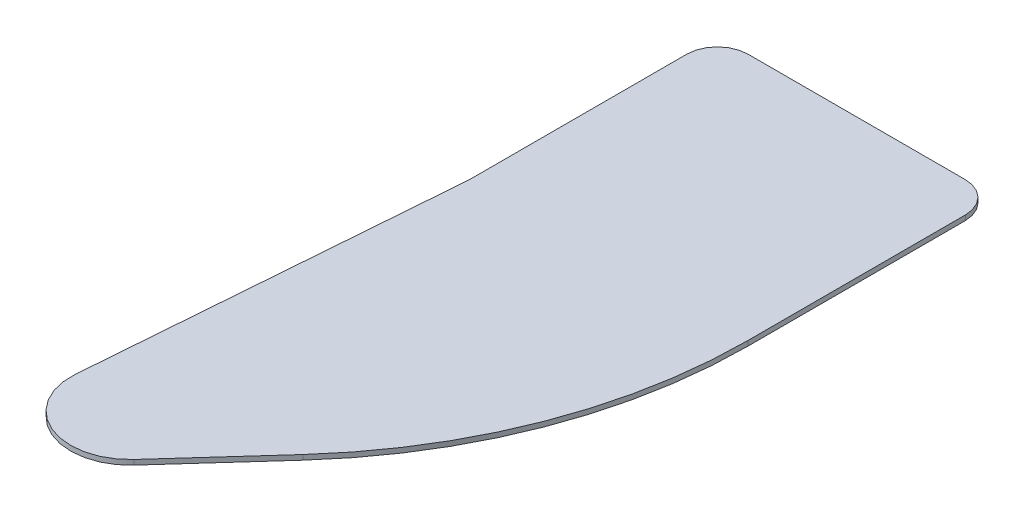
# Autodesk Inventor part: m2stack_bottom_1
Saved by Autodesk Inventor 2026 (Build 300175000, 175)
## iProperties
Created: 2025-05-07
Part Number: m2stack_bottom_1
Material: Generic
Document SubType Name: Modeling
Designer: Paul Juschitz
Density: 1 g/cm^3
Appearance: Default
Author: Paul Juschitz
Autodesk Inventor part; units mm, degrees
ref_plane "YZ Plane" through (0, 0, 0) normal (1, 0, 0) x (0, 1, 0)
ref_plane "XZ Plane" through (0, 0, 0) normal (0, 1, 0) x (-1, 0, 0)
ref_plane "XY Plane" through (0, 0, 0) normal (0, 0, 1) x (1, 0, 0)
sketch "Sketch1" plane through (0, 0, 0) normal (0, 1, 0) x (-1, 0, 0)
  line L0 (50, 0) -> (-50, 0)
  line L1 (0, 50) -> (0, -50)
  line L2 (-25.0156, 15.5413) -> (-25.0156, -28.4587)
  arc A0 (-25.0156, -28.4587) -> (-18.8156, -34.6587) centre (-18.8156, -28.4587) ccw
  line L3 (-18.8156, -34.6587) -> (25.1844, -34.6587)
  arc A1 (25.1844, -34.6587) -> (31.3844, -28.4587) centre (25.1844, -28.4587) ccw
  line L4 (31.3844, -28.4587) -> (31.3844, 15.5413)
  line L5 (31.3844, 15.5413) -> (37.1483, 89.6103)
  arc A2 (37.1483, 89.6103) -> (16.2805, 98.5862) centre (25.1844, 90.5413) ccw
  line L6 (16.2805, 98.5862) -> (0.0171, 80.5862)
  arc A3 (0.0171, 80.5862) -> (-25.0156, 15.5413) centre (72.0072, 15.5413) ccw
  line L7 (31.3844, 15.5413) -> (-25.0156, 15.5413) construction
  point P0 (0, 0)
  point P1 (31.3844, 15.5413)
  dimension "d0" = 100
  dimension "d1" = 100
  dimension "d3" = 56.4
  dimension "d4" = 6.2
  dimension "case_foot_outer_radius" = 12
  dimension "case_foot_width" = 75
  dimension "d7" = 18
  constraints: 16 end point, 8 point on circle, 8 tangent, 4 centre point, 3 perpendicular, 3 vertical, 2 equal length, 2 midpoint, 1 coincident, 1 equal radius, 1 horizontal, 1 vertical alignment, 6 other
  measures "d0" distance of L0.start L0.end
  measures "d1" distance of L1.start L1.end
  measures "d3" distance between parallel lines of L2 L4
  measures "d4" radius of A0
  measures "case_foot_outer_radius" radius of A2
  measures "case_foot_width" distance from line of L7 A2.centre
  measures "d7" vertical distance of L6.end L6.start
extrude "Extrusion1" add sketch "Sketch1" along normal blind 1
equation "\"d3\" = core_outer_width + 2 * case_spacing + 2 * case_thickness"
equation "\"d4\" = core_outer_radius + case_thickness + case_spacing"
equation "\"case_spacing\" = 0.2"
equation "\"core_outer_width\" = 54"
equation "\"case_thickness\" = 1"
equation "\"core_outer_radius\" = 5"
body "Solid1"
